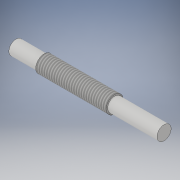
# Autodesk Inventor part: Small Gear Shaft
Saved by Autodesk Inventor 2019 (Build 230136000, 136)
## iProperties
Created: 2021-06-06
Part Number: Small Gear Shaft
Material: Generic
Document SubType Name: Modeling
Designer: micha
Density: 1 g/cm^3
Appearance: Default
Author: micha
Autodesk Inventor part; units mm, degrees
ref_plane "YZ Plane" through (0, 0, 0) normal (1, 0, 0) x (0, 1, 0)
ref_plane "XZ Plane" through (0, 0, 0) normal (0, 1, 0) x (-1, 0, 0)
ref_plane "XY Plane" through (0, 0, 0) normal (0, 0, 1) x (1, 0, 0)
sketch "Sketch1" plane through (0, 0, 0) normal (0, 0, 1) x (1, 0, 0)
  line L0 (0, 0) -> (85, 0)
  line L1 (0, 6) -> (0, 0)
  line L2 (50, 6) -> (50, 5)
  line L3 (50, 5) -> (85, 5)
  line L4 (85, 5) -> (85, 0)
  line L5 (50, 6) -> (0, 6)
  line L6 (0, 6) -> (0, 5)
  line L7 (0, 5) -> (-20, 5)
  line L8 (-20, 5) -> (-20, 0)
  line L9 (-20, 0) -> (0, 0)
  dimension "d10" = 1
  dimension "d11" = 35
  dimension "d12" = 5
  dimension "d16" = 20
  dimension "d17" = 5
  dimension "d18" = 50
  constraints: 20 end point, 4 perpendicular, 3 horizontal, 2 vertical, 1 point on line
  measures "d10" distance of L2.start L2.end
  measures "d11" distance of L2.end L3.end
  measures "d12" distance of L3.end L0.end
  measures "d16" distance of L6.end L7.end
  measures "d17" distance of L7.end L8.end
  measures "d18" distance of L2.start L1.start
revolve "Revolution1" add sketch "Sketch1" angle 360 about axis through (0, 0, 0) along (1, 0, 0)
thread "Thread2" size "M12x1.75" class "6g" standard "ANSI Metric M Profile" full length
body "Solid1"
